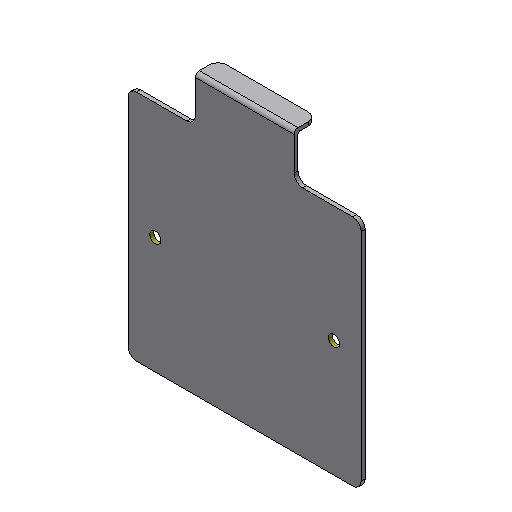
# Autodesk Inventor part: TL20240701-10110CV-025
Saved by Autodesk Inventor 2022.5 (Build 265521000, 521)
## iProperties
Category: DRIVE UNIT ASSY
Company: 현대 트랜시스(대유)
RuleStatus: InUse
Created: 2023-05-11
Part Number: TL20240701-10110CV-025
Checked By: 김형민
Engr Approved By: 김시현
User Status: 1 x18
Material: SS400
Description: 0
Document SubType Name: Modeling
Mfg Approved By: 호상태
Designer: 김건휴
Stock Number: 025
Density: 7.85 g/cm^3
Appearance: Painting-RAL7035
Project: SW PJT
BeforeDocSave0: file://D:\V\Templates\iLogic\PART\Part Design STD iLogic
DETAIL: Coveryor Assembly
M/C TITLE: CJ 제일제당 협동로봇 포장시스탬 PILOT 장비
PARTS NAME: Bracket
SPECIFICATION: TA20221101-CV200000-015
DocNumber: 221118_Standard_v1
Folder: .\
VDS_Category: 엔지니어링
Detail Description: Processed products
Title: COVER
Subject: SW차종 시트조립라인
Author: 김건휴
Revision Number: A
Autodesk Inventor part; units mm, degrees
ref_plane "YZ Plane" through (0, 0, 0) normal (1, 0, 0) x (0, 1, 0)
ref_plane "XZ Plane" through (0, 0, 0) normal (0, 1, 0) x (-1, 0, 0)
ref_plane "XY Plane" through (0, 0, 0) normal (0, 0, 1) x (1, 0, 0)
sketch "스케치9" plane through (0, 0, 0) normal (0, 0, 1) x (1, 0, 0)
  line L0 (-68.5, 68.5) -> (68.5, 68.5)
  line L1 (68.5, 68.5) -> (68.5, -68.5)
  line L2 (68.5, -68.5) -> (-68.5, -68.5)
  line L3 (-68.5, -68.5) -> (-68.5, 68.5)
  line L4 (-68.5, 68.5) -> (68.5, -68.5) construction
  line L5 (68.5, 68.5) -> (-68.5, -68.5) construction
  line L6 (-29, 95.5) -> (29, 95.5)
  line L7 (29, 95.5) -> (29, 41.5)
  line L8 (29, 41.5) -> (-29, 41.5)
  line L9 (-29, 41.5) -> (-29, 95.5)
  line L10 (-29, 95.5) -> (29, 41.5) construction
  line L11 (29, 95.5) -> (-29, 41.5) construction
  point P0 (0, 0)
  point P1 (0, 68.5)
  point P2 (29, 68.5)
  point P3 (-29, 68.5)
  dimension "d40" = 137
  dimension "d41" = 137
  dimension "d42" = 58
  dimension "d43" = 27
  constraints: 24 end point, 5 midpoint, 4 parallel, 2 horizontal, 2 perpendicular
  measures "d40" distance of L0.start L0.end
  measures "d41" distance of L0.end L1.end
  measures "d42" distance between parallel lines of L7 L9
  measures "d43" distance between parallel lines of L0 L6
extrude "돌출4" add sketch "스케치9" along normal mid plane 2.3
sketch "스케치10" plane through (0, 0, -1.15) normal (0, 0, -1) x (-1, 0, 0)
  line L0 (-29, 68.5) -> (-29, 95.5) projected
  line L1 (29, 95.5) -> (29, 68.5) projected
  line L2 (-29, 95.5) -> (29, 95.5)
  line L3 (29, 95.5) -> (29, 93.2)
  line L4 (29, 93.2) -> (-29, 93.2)
  line L5 (-29, 93.2) -> (-29, 95.5)
  point P0 (0, 0)
  point P1 (-29, 93.2)
  dimension "d46" = 2.3
  constraints: 8 end point, 2 parallel, 1 horizontal, 1 perpendicular, 1 point on line
  measures "d46" distance between parallel lines of L4 L2
extrude "돌출5" add sketch "스케치10" along normal blind 11
fillet "모깎기2" radius 5 6 edges at (68.5, 68.5, 0) (-68.5, 68.5, 0) (68.5, -68.5, 0) (-68.5, -68.5, 0) (29, 94.35, -12.15) (-29, 94.35, -12.15)
sketch "스케치11" plane through (0, 0, 1.15) normal (0, 0, 1) x (1, 0, 0)
  line L0 (-68.5, 63.5) -> (-68.5, -63.5) projected
  line L1 (63.5, 68.5) -> (29, 68.5) projected
  point P0 (0, 0)
  point P1 (52.5, 0)
  point P2 (-52.5, 0)
  dimension "d50" = 105
  dimension "d52" = 16
  constraints: 2 horizontal alignment
  measures "d50" distance of point (52.5, 0) point (-52.5, 0)
  measures "d52" distance from line of point (-52.5, 0) L0
hole "구멍3" at (52.5, 0, 1.15) at (-52.5, 0, 1.15) direction (0, 0, -1) diameter 6.6 end through all clearance for "Socket Head Cap Screw" size "M6" standard "TS Profile"
fillet "모깎기3" radius 1.15 1 edges at (0, 93.2, -1.15)
fillet "모깎기3" radius 2.3 1 edges at (0, 95.5, 1.15)
fillet "모깎기5" radius 5 2 edges at (29, 68.5, 0) (-29, 68.5, 0)
equation "\"d61\" = 0.5 * d44"
equation "\"d64\" = d44"
equation "\"d44\" = 2.3"
